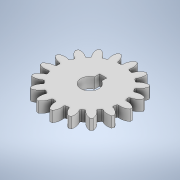
# Autodesk Inventor part: Fixed_gear
Saved by Autodesk Inventor 2020 (Build 240168000, 168)
## iProperties
Created: 2020-05-11
Part Number: Fixed_gear
Material: Generic
Document SubType Name: Modeling
Designer: avi41
Density: 1 g/cm^3
Appearance: Default
Author: avi41
Autodesk Inventor part; units mm, degrees
ref_plane "YZ Plane" through (0, 0, 0) normal (1, 0, 0) x (0, 1, 0)
ref_plane "XZ Plane" through (0, 0, 0) normal (0, 1, 0) x (-1, 0, 0)
ref_plane "XY Plane" through (0, 0, 0) normal (0, 0, 1) x (1, 0, 0)
sketch "Sketch1" plane through (0, 0, 0) normal (0, 1, 0) x (-1, 0, 0)
  arc A0 (0.3488, -8.9491) -> (-2.2796, -8.6609) centre (0, 0) ccw construction
  line L0 (0, -21.7523) -> (0, 17.3166) construction
  line L1 (-16.4294, 0) -> (16.4294, 0) construction
  arc A1 (0.3488, -8.9491) -> (-2.2796, -8.6609) centre (0, 0) ccw
  circle A2 centre (0, 0) radius 11.7353 construction
  circle A3 centre (0, 0) radius 10.5 construction
  line L2 (0, 0) -> (-4.0137, -11.0276) construction
  circle A4 centre (0, 0) radius 9.8668 construction
  line L3 (-3.3746, -9.2717) -> (5.3254, -12.4383) construction
  line L4 (3.5046, -9.8668) -> (-4.0266, -9.8668) construction
  arc A5 (-0.9533, -11.6965) -> (0.052, -9.2588) centre (-3.3746, -9.2717) ccw
  circle A6 centre (0, 0) radius 9.2647 construction
  arc A7 (0.3488, -8.9491) -> (0.052, -9.2588) centre (0.3609, -9.2577) ccw
  line L5 (-1.3339, -12.1661) -> (-0.7958, -7.2586) construction
  arc A8 (-2.057, -9.0276) -> (-1.6037, -11.6252) centre (1.2855, -9.7827) ccw
  arc A9 (-2.057, -9.0276) -> (-2.2796, -8.6609) centre (-2.3582, -8.9595) ccw
  line L6 (-0.9533, -11.6965) -> (-1.6037, -11.6252)
  point P0 (0, -9.8668)
  point P1 (-0.149, -9.2635)
  point P2 (0, -16.1711)
  point P3 (-0.1751, -10.4985)
  point P4 (-1.8617, -9.0757)
  point P5 (-3.504, -15.7869)
  point P6 (-0.1601, -15.8391)
  point P7 (-6.1857, -13.0529)
  point P8 (-5.7886, -14.7444)
  point P9 (-1.2807, -6.5842)
  dimension "d23" = 21
  dimension "d25" = 1.5441
  dimension "d26" = 1.2353
  dimension "d27" = 20
  dimension "d28" = 19.7336
  dimension "d29" = 20
  dimension "d30" = 0.3088
  dimension "d31" = 0.6177
  dimension "d32" = 0.9702
  constraints: 18 point on circle, 10 end point, 8 centre point, 7 coincident, 6 symmetric about line, 4 point on line, 3 tangent, 1 concentric, 1 horizontal, 8 other
  measures "d27" angle of L0 L2
  measures "d28" diameter of A4
  measures "d29" angle of L4 L3
  measures "d31" diameter of A7
  measures "d32" distance from line of point (-0.175, -10.499) L5
extrude "Extrusion1" add sketch "Sketch1" along normal mid plane 3
pattern_circular "Circular Pattern2" count 17 over 360 about axis through (0, -10, 0) along (0, 1, 0) of "Extrusion1"
sketch "Sketch2" plane through (0, 1.5, 0) normal (0, 1, 0) x (1, 0, 0)
  arc A0 (-1, 2.2913) -> (1, 2.2913) centre (0, 0) ccw
  line L0 (-1, 2.2913) -> (-1, 3.7)
  line L1 (-1, 3.7) -> (1, 3.7)
  line L2 (1, 3.7) -> (1, 2.2913)
  line L3 (0, 15.827) -> (0, -13.0864) construction
  dimension "d13" = 5
  dimension "d14" = 2
  dimension "d15" = 3.7
  constraints: 6 end point, 2 perpendicular, 2 point on circle, 1 centre point, 1 coincident, 1 vertical, 1 other
  measures "d13" diameter of A0
  measures "d14" distance of L0.end L1.end
  measures "d15" distance from line of point (0, 0) L1
extrude "Extrusion2" cut sketch "Sketch2" against normal through all
equation "\"d23\" = pitch_diam"
equation "\"d25\" = dedendum"
equation "\"d26\" = addendum"
equation "\"d27\" = pressure_ang"
equation "\"d28\" = 2 * base_circ"
equation "\"d29\" = pressure_ang"
equation "\"d30\" = clearance"
equation "\"d31\" = 2 * fillet_r"
equation "\"d32\" = 0.5 * thickness_tooth"
equation "\"pitch_diam\" = 21"
equation "\"clearance\" = dedendum - addendum"
equation "\"addendum\" = module"
equation "\"dedendum\" = 1.25 * module"
equation "\"fillet_r\" = clearance"
equation "\"thickness_tooth\" = 0.5 * pitch_circ"
equation "\"pitch_circ\" = 3.1416 * module"
equation "\"pressure_ang\" = 20deg"
equation "\"base_circ\" = 9.866773"
equation "\"module\" = 1.235294"
body "Solid1"
